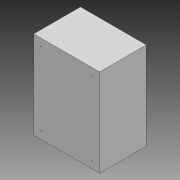
# Autodesk Inventor part: Part38
Saved by Autodesk Inventor 2018 (Build 220112000, 112)
## iProperties
Created: 2022-04-21
Part Number: Part38
Material: Generic
Document SubType Name: Modeling
Designer: pollak
Density: 1 g/cm^3
Appearance: Default
Author: pollak
Autodesk Inventor part; units mm, degrees
ref_plane "YZ Plane" through (0, 0, 0) normal (1, 0, 0) x (0, 1, 0)
ref_plane "XZ Plane" through (0, 0, 0) normal (0, 1, 0) x (-1, 0, 0)
ref_plane "XY Plane" through (0, 0, 0) normal (0, 0, 1) x (1, 0, 0)
sketch "Sketch1" plane through (0, 0, 0) normal (0, 1, 0) x (-1, 0, 0)
  line L0 (114.3, 152.4) -> (-114.3, 152.4)
  line L1 (-114.3, 152.4) -> (-114.3, -152.4)
  line L2 (-114.3, -152.4) -> (114.3, -152.4)
  line L3 (114.3, -152.4) -> (114.3, 152.4)
  line L4 (114.3, 152.4) -> (-114.3, -152.4) construction
  line L5 (-114.3, 152.4) -> (114.3, -152.4) construction
  point P0 (0, 0)
  dimension "d0" = 228.6
  dimension "d1" = 304.8
  constraints: 12 end point, 2 midpoint, 2 parallel, 1 horizontal, 1 perpendicular
  measures "d0" distance of L2.end L1.end
  measures "d1" distance of L1.end L0.end
extrude "Extrusion1" add sketch "Sketch1" along normal blind 2.5
sketch "Sketch2" plane through (0, 2.5, 0) normal (0, 1, 0) x (1, 0, 0)
  line L0 (114.3, 152.4) -> (-114.3, 152.4) projected
  line L1 (-114.3, -152.4) -> (114.3, -152.4)
  line L2 (114.3, -152.4) -> (114.3, 152.4)
  line L3 (114.3, 152.4) -> (-114.3, 152.4)
  line L4 (-114.3, 152.4) -> (-114.3, -152.4)
  line L5 (-114.3, -152.4) -> (114.3, 152.4) construction
  line L6 (114.3, -152.4) -> (-114.3, 152.4) construction
  line L7 (-112.3, -150.4) -> (112.3, -150.4)
  line L8 (112.3, -150.4) -> (112.3, 150.4)
  line L9 (112.3, 150.4) -> (-112.3, 150.4)
  line L10 (-112.3, 150.4) -> (-112.3, -150.4)
  line L11 (-112.3, -150.4) -> (112.3, 150.4) construction
  line L12 (112.3, -150.4) -> (-112.3, 150.4) construction
  point P0 (0, 0)
  dimension "d4" = 2
  dimension "d5" = 2
  constraints: 24 end point, 4 midpoint, 4 parallel, 2 horizontal, 2 perpendicular
  measures "d4" distance between parallel lines of L4 L10
  measures "d5" distance between parallel lines of L0 L9
extrude "Extrusion2" add sketch "Sketch2" along normal blind 145
sketch "Sketch3" plane through (0, 147.5, 0) normal (0, 1, 0) x (1, 0, 0)
  line L0 (114.3, -152.4) -> (114.3, 152.4) projected
  line L1 (-114.3, -152.4) -> (114.3, -152.4)
  line L2 (114.3, -152.4) -> (114.3, 152.4)
  line L3 (114.3, 152.4) -> (-114.3, 152.4)
  line L4 (-114.3, 152.4) -> (-114.3, -152.4)
  line L5 (-114.3, -152.4) -> (114.3, 152.4) construction
  line L6 (114.3, -152.4) -> (-114.3, 152.4) construction
  line L7 (-99.3, -137.4) -> (99.3, -137.4)
  line L8 (99.3, -137.4) -> (99.3, 137.4)
  line L9 (99.3, 137.4) -> (-99.3, 137.4)
  line L10 (-99.3, 137.4) -> (-99.3, -137.4)
  line L11 (-99.3, -137.4) -> (99.3, 137.4) construction
  line L12 (99.3, -137.4) -> (-99.3, 137.4) construction
  point P0 (0, 0)
  dimension "d8" = 15
  dimension "d9" = 15
  constraints: 24 end point, 4 midpoint, 4 parallel, 2 horizontal, 2 perpendicular
  measures "d8" distance between parallel lines of L4 L10
  measures "d9" distance between parallel lines of L3 L9
extrude "Extrusion3" add sketch "Sketch3" along normal blind 15
sketch "Sketch4" plane through (-112.3, 2.5, -150.4) normal (0, 0, 1) x (1, 0, 0)
  line L0 (78.3, 108) -> (146.3, 108)
  line L1 (146.3, 108) -> (146.3, 84)
  line L2 (146.3, 84) -> (78.3, 84)
  line L3 (78.3, 84) -> (78.3, 108)
  line L4 (78.3, 108) -> (146.3, 84) construction
  line L5 (146.3, 108) -> (78.3, 84) construction
  line L6 (13, 160) -> (211.6, 160) projected
  line L7 (0, 0) -> (0, 145) projected
  line L8 (226.6, -2.5) -> (226.6, 160) projected
  point P0 (112.3, -2.5)
  point P1 (112.3, 96)
  dimension "d12" = 68
  dimension "d13" = 24
  dimension "d14" = 52
  dimension "d17" = 80.3
  constraints: 12 end point, 2 midpoint, 2 parallel, 1 horizontal, 1 perpendicular
  measures "d12" distance of L1.end L2.end
  measures "d13" distance of L0.end L1.end
  measures "d14" distance between parallel lines of L0 L6
  measures "d17" distance between parallel lines of L8 L1
extrude "Extrusion4" add sketch "Sketch4" along normal blind 40
sketch "Sketch5" plane through (0, 0, 0) normal (0, -1, 0) x (1, 0, 0)
  line L0 (88.9, -127) -> (-88.9, -127) construction
  line L1 (-88.9, -127) -> (-88.9, 127) construction
  line L2 (-88.9, 127) -> (88.9, 127) construction
  line L3 (88.9, 127) -> (88.9, -127) construction
  line L4 (88.9, -127) -> (-88.9, 127) construction
  line L5 (-88.9, -127) -> (88.9, 127) construction
  point P0 (0, 0)
  dimension "d20" = 177.8
  dimension "d21" = 254
  constraints: 12 end point, 4 coincident, 2 midpoint, 2 parallel, 1 horizontal, 1 perpendicular
  measures "d20" distance of L1.end L2.end
  measures "d21" distance of L0.end L1.end
hole "Hole1" at (88.9, 0, -127) at (88.9, 0, 127) at (-88.9, 0, 127) at (-88.9, 0, -127) direction (0, 1, 0) diameter 3.302 end through all thread size "8-32 UNC" class "2B" standard "ANSI Unified Screw Threads"
body "Solid1"
